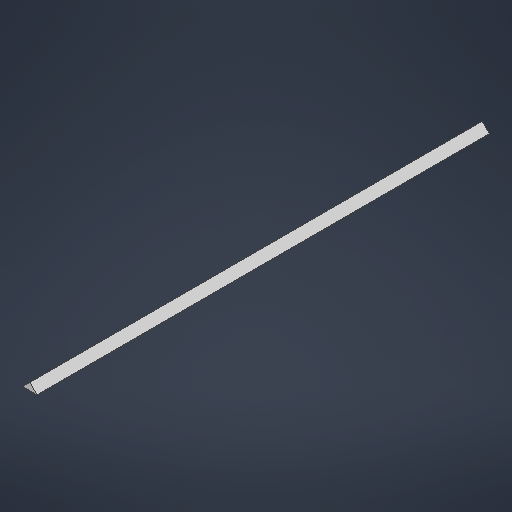
# Autodesk Inventor part: CoinActivator
Saved by Autodesk Inventor 2026.3 (Build 303398000, 398)
## iProperties
Created: 2026-05-07
Part Number: CoinActivator
Material: Generic
Document SubType Name: Modeling
Designer: frede
Density: 1 g/cm^3
Appearance: Default
Author: frede
Autodesk Inventor part; units mm, degrees
ref_plane "YZ Plane" through (0, 0, 0) normal (1, 0, 0) x (0, 1, 0)
ref_plane "XZ Plane" through (0, 0, 0) normal (0, 1, 0) x (-1, 0, 0)
ref_plane "XY Plane" through (0, 0, 0) normal (0, 0, 1) x (1, 0, 0)
sketch "Sketch1" plane through (0, 0, 0) normal (0, 0, 1) x (1, 0, 0)
  line L0 (0, 0) -> (4, 0)
  line L1 (2, 0) -> (2, 2)
  line L2 (2, 2) -> (0, 0)
  line L3 (2, 2) -> (4, 0)
  dimension "d1" = 90
  dimension "d2" = 2
  constraints: 8 end point, 1 horizontal, 1 midpoint, 1 perpendicular
  measures "d1" angle of L3 L2
  measures "d2" distance of L1.start L1.end
extrude "Extrusion1" add sketch "Sketch1" along normal blind 126
body "Solid1"
